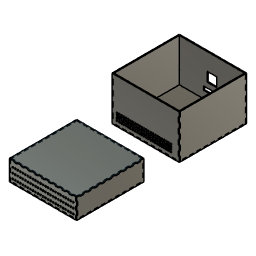
Boite projetV2 v3 (Autodesk Fusion 360 design; units mm, degrees)
Autodesk Fusion 360 part; units mm, degrees
(part 1 of 3)
sketch "Esquisse1" plane through (0, 0, 0) normal (0, 0, 1) x (1, 0, 0)
sketch "Esquisse2" plane through (0, 0, 0) normal (0, 0, 1) x (1, 0, 0)
  line L0 (0, 0) -> (200, 0)
  line L1 (200, 0) -> (200, 200)
  line L2 (200, 200) -> (0, 200)
  line L3 (0, 200) -> (0, 0)
  line L4 (0, 0) -> (10.5263, 0)
  line L5 (10.5263, 0) -> (10.5263, 3)
  line L6 (10.5263, 3) -> (0, 3)
  line L7 (0, 3) -> (0, 0)
  line L8 (10.5263, 0) -> (21.0526, 0)
  line L9 (21.0526, 0) -> (21.0526, 3)
  line L10 (21.0526, 3) -> (10.5263, 3)
  line L11 (10.5263, 3) -> (10.5263, 0)
  line L12 (21.0526, 0) -> (31.5789, 0)
  line L13 (31.5789, 0) -> (31.5789, 3)
  line L14 (31.5789, 3) -> (21.0526, 3)
  line L15 (21.0526, 3) -> (21.0526, 0)
  line L16 (31.5789, 0) -> (42.1053, 0)
  line L17 (42.1053, 0) -> (42.1053, 3)
  line L18 (42.1053, 3) -> (31.5789, 3)
  line L19 (31.5789, 3) -> (31.5789, 0)
  line L20 (42.1053, 0) -> (52.6316, 0)
  line L21 (52.6316, 0) -> (52.6316, 3)
  line L22 (52.6316, 3) -> (42.1053, 3)
  line L23 (42.1053, 3) -> (42.1053, 0)
  line L24 (52.6316, 0) -> (63.1579, 0)
  line L25 (63.1579, 0) -> (63.1579, 3)
  line L26 (63.1579, 3) -> (52.6316, 3)
  line L27 (52.6316, 3) -> (52.6316, 0)
  line L28 (63.1579, 0) -> (73.6842, 0)
  line L29 (73.6842, 0) -> (73.6842, 3)
  line L30 (73.6842, 3) -> (63.1579, 3)
  line L31 (63.1579, 3) -> (63.1579, 0)
  line L32 (73.6842, 0) -> (84.2105, 0)
  line L33 (84.2105, 0) -> (84.2105, 3)
  line L34 (84.2105, 3) -> (73.6842, 3)
  line L35 (73.6842, 3) -> (73.6842, 0)
  line L36 (84.2105, 0) -> (94.7368, 0)
  line L37 (94.7368, 0) -> (94.7368, 3)
  line L38 (94.7368, 3) -> (84.2105, 3)
  line L39 (84.2105, 3) -> (84.2105, 0)
  line L40 (94.7368, 0) -> (105.2632, 0)
  line L41 (105.2632, 0) -> (105.2632, 3)
  line L42 (105.2632, 3) -> (94.7368, 3)
  line L43 (94.7368, 3) -> (94.7368, 0)
  line L44 (105.2632, 0) -> (115.7895, 0)
  line L45 (115.7895, 0) -> (115.7895, 3)
  line L46 (115.7895, 3) -> (105.2632, 3)
  line L47 (105.2632, 3) -> (105.2632, 0)
  line L48 (115.7895, 0) -> (126.3158, 0)
  line L49 (126.3158, 0) -> (126.3158, 3)
  line L50 (126.3158, 3) -> (115.7895, 3)
  line L51 (115.7895, 3) -> (115.7895, 0)
  line L52 (126.3158, 0) -> (136.8421, 0)
  line L53 (136.8421, 0) -> (136.8421, 3)
  line L54 (136.8421, 3) -> (126.3158, 3)
  line L55 (126.3158, 3) -> (126.3158, 0)
  line L56 (136.8421, 0) -> (147.3684, 0)
  line L57 (147.3684, 0) -> (147.3684, 3)
  line L58 (147.3684, 3) -> (136.8421, 3)
  line L59 (136.8421, 3) -> (136.8421, 0)
  line L60 (147.3684, 0) -> (157.8947, 0)
  line L61 (157.8947, 0) -> (157.8947, 3)
  line L62 (157.8947, 3) -> (147.3684, 3)
  line L63 (147.3684, 3) -> (147.3684, 0)
  line L64 (157.8947, 0) -> (168.4211, 0)
  line L65 (168.4211, 0) -> (168.4211, 3)
  line L66 (168.4211, 3) -> (157.8947, 3)
  line L67 (157.8947, 3) -> (157.8947, 0)
  line L68 (168.4211, 0) -> (178.9474, 0)
  line L69 (178.9474, 0) -> (178.9474, 3)
  line L70 (178.9474, 3) -> (168.4211, 3)
  line L71 (168.4211, 3) -> (168.4211, 0)
  line L72 (178.9474, 0) -> (189.4737, 0)
  line L73 (189.4737, 0) -> (189.4737, 3)
  line L74 (189.4737, 3) -> (178.9474, 3)
  line L75 (178.9474, 3) -> (178.9474, 0)
  line L76 (189.4737, 0) -> (200, 0)
  line L77 (200, 0) -> (200, 3)
  line L78 (200, 3) -> (189.4737, 3)
  line L79 (189.4737, 3) -> (189.4737, 0)
  line L80 (0, 197) -> (10.5263, 197)
  line L81 (10.5263, 197) -> (10.5263, 200)
  line L82 (10.5263, 200) -> (0, 200)
  line L83 (0, 200) -> (0, 197)
  line L84 (10.5263, 197) -> (21.0526, 197)
  line L85 (21.0526, 197) -> (21.0526, 200)
  line L86 (21.0526, 200) -> (10.5263, 200)
  line L87 (10.5263, 200) -> (10.5263, 197)
  line L88 (21.0526, 197) -> (31.5789, 197)
  line L89 (31.5789, 197) -> (31.5789, 200)
  line L90 (31.5789, 200) -> (21.0526, 200)
  line L91 (21.0526, 200) -> (21.0526, 197)
  line L92 (31.5789, 197) -> (42.1053, 197)
  line L93 (42.1053, 197) -> (42.1053, 200)
  line L94 (42.1053, 200) -> (31.5789, 200)
  line L95 (31.5789, 200) -> (31.5789, 197)
  line L96 (42.1053, 197) -> (52.6316, 197)
  line L97 (52.6316, 197) -> (52.6316, 200)
  line L98 (52.6316, 200) -> (42.1053, 200)
  line L99 (42.1053, 200) -> (42.1053, 197)
  line L100 (52.6316, 197) -> (63.1579, 197)
  line L101 (63.1579, 197) -> (63.1579, 200)
  line L102 (63.1579, 200) -> (52.6316, 200)
  line L103 (52.6316, 200) -> (52.6316, 197)
  line L104 (63.1579, 197) -> (73.6842, 197)
  line L105 (73.6842, 197) -> (73.6842, 200)
  line L106 (73.6842, 200) -> (63.1579, 200)
  line L107 (63.1579, 200) -> (63.1579, 197)
  line L108 (73.6842, 197) -> (84.2105, 197)
  line L109 (84.2105, 197) -> (84.2105, 200)
  line L110 (84.2105, 200) -> (73.6842, 200)
  line L111 (73.6842, 200) -> (73.6842, 197)
  line L112 (84.2105, 197) -> (94.7368, 197)
  line L113 (94.7368, 197) -> (94.7368, 200)
  line L114 (94.7368, 200) -> (84.2105, 200)
  line L115 (84.2105, 200) -> (84.2105, 197)
  line L116 (94.7368, 197) -> (105.2632, 197)
  line L117 (105.2632, 197) -> (105.2632, 200)
  line L118 (105.2632, 200) -> (94.7368, 200)
  line L119 (94.7368, 200) -> (94.7368, 197)
  line L120 (105.2632, 197) -> (115.7895, 197)
  line L121 (115.7895, 197) -> (115.7895, 200)
  line L122 (115.7895, 200) -> (105.2632, 200)
  line L123 (105.2632, 200) -> (105.2632, 197)
  line L124 (115.7895, 197) -> (126.3158, 197)
  line L125 (126.3158, 197) -> (126.3158, 200)
  line L126 (126.3158, 200) -> (115.7895, 200)
  line L127 (115.7895, 200) -> (115.7895, 197)
  line L128 (126.3158, 197) -> (136.8421, 197)
  line L129 (136.8421, 197) -> (136.8421, 200)
  line L130 (136.8421, 200) -> (126.3158, 200)
  line L131 (126.3158, 200) -> (126.3158, 197)
  line L132 (136.8421, 197) -> (147.3684, 197)
  line L133 (147.3684, 197) -> (147.3684, 200)
  line L134 (147.3684, 200) -> (136.8421, 200)
  line L135 (136.8421, 200) -> (136.8421, 197)
  line L136 (147.3684, 197) -> (157.8947, 197)
  line L137 (157.8947, 197) -> (157.8947, 200)
  line L138 (157.8947, 200) -> (147.3684, 200)
  line L139 (147.3684, 200) -> (147.3684, 197)
  line L140 (157.8947, 197) -> (168.4211, 197)
  line L141 (168.4211, 197) -> (168.4211, 200)
  line L142 (168.4211, 200) -> (157.8947, 200)
  line L143 (157.8947, 200) -> (157.8947, 197)
  line L144 (168.4211, 197) -> (178.9474, 197)
  line L145 (178.9474, 197) -> (178.9474, 200)
  line L146 (178.9474, 200) -> (168.4211, 200)
  line L147 (168.4211, 200) -> (168.4211, 197)
  line L148 (178.9474, 197) -> (189.4737, 197)
  line L149 (189.4737, 197) -> (189.4737, 200)
  line L150 (189.4737, 200) -> (178.9474, 200)
  line L151 (178.9474, 200) -> (178.9474, 197)
  line L152 (189.4737, 197) -> (200, 197)
  line L153 (200, 197) -> (200, 200)
  line L154 (200, 200) -> (189.4737, 200)
  line L155 (189.4737, 200) -> (189.4737, 197)
  line L156 (0, 0) -> (3, 0)
  line L157 (3, 0) -> (3, 10.5263)
  line L158 (3, 10.5263) -> (0, 10.5263)
  line L159 (0, 10.5263) -> (0, 0)
  line L160 (197, 10.5263) -> (197, 0)
  line L161 (197, 0) -> (200, 0)
  line L162 (200, 0) -> (200, 10.5263)
  line L163 (200, 10.5263) -> (197, 10.5263)
  line L164 (0, 21.0526) -> (0, 10.5263)
  line L165 (0, 10.5263) -> (3, 10.5263)
  line L166 (3, 10.5263) -> (3, 21.0526)
  line L167 (3, 21.0526) -> (0, 21.0526)
  line L168 (197, 21.0526) -> (197, 10.5263)
  line L169 (197, 10.5263) -> (200, 10.5263)
  line L170 (200, 10.5263) -> (200, 21.0526)
  line L171 (200, 21.0526) -> (197, 21.0526)
  line L172 (0, 31.5789) -> (0, 21.0526)
  line L173 (0, 21.0526) -> (3, 21.0526)
  line L174 (3, 21.0526) -> (3, 31.5789)
  line L175 (3, 31.5789) -> (0, 31.5789)
  line L176 (197, 31.5789) -> (197, 21.0526)
  line L177 (197, 21.0526) -> (200, 21.0526)
  line L178 (200, 21.0526) -> (200, 31.5789)
  line L179 (200, 31.5789) -> (197, 31.5789)
  line L180 (0, 42.1053) -> (0, 31.5789)
  line L181 (0, 31.5789) -> (3, 31.5789)
  line L182 (3, 31.5789) -> (3, 42.1053)
  line L183 (3, 42.1053) -> (0, 42.1053)
  line L184 (197, 42.1053) -> (197, 31.5789)
  line L185 (197, 31.5789) -> (200, 31.5789)
  line L186 (200, 31.5789) -> (200, 42.1053)
  line L187 (200, 42.1053) -> (197, 42.1053)
  line L188 (0, 52.6316) -> (0, 42.1053)
  line L189 (0, 42.1053) -> (3, 42.1053)
  line L190 (3, 42.1053) -> (3, 52.6316)
  line L191 (3, 52.6316) -> (0, 52.6316)
  line L192 (197, 52.6316) -> (197, 42.1053)
  line L193 (197, 42.1053) -> (200, 42.1053)
  line L194 (200, 42.1053) -> (200, 52.6316)
  line L195 (200, 52.6316) -> (197, 52.6316)
  line L196 (0, 63.1579) -> (0, 52.6316)
  line L197 (0, 52.6316) -> (3, 52.6316)
  line L198 (3, 52.6316) -> (3, 63.1579)
  line L199 (3, 63.1579) -> (0, 63.1579)
  line L200 (197, 63.1579) -> (197, 52.6316)
  line L201 (197, 52.6316) -> (200, 52.6316)
  line L202 (200, 52.6316) -> (200, 63.1579)
  line L203 (200, 63.1579) -> (197, 63.1579)
  line L204 (0, 73.6842) -> (0, 63.1579)
  line L205 (0, 63.1579) -> (3, 63.1579)
  line L206 (3, 63.1579) -> (3, 73.6842)
  line L207 (3, 73.6842) -> (0, 73.6842)
  line L208 (197, 73.6842) -> (197, 63.1579)
  line L209 (197, 63.1579) -> (200, 63.1579)
  line L210 (200, 63.1579) -> (200, 73.6842)
  line L211 (200, 73.6842) -> (197, 73.6842)
  line L212 (0, 84.2105) -> (0, 73.6842)
  line L213 (0, 73.6842) -> (3, 73.6842)
  line L214 (3, 73.6842) -> (3, 84.2105)
  line L215 (3, 84.2105) -> (0, 84.2105)
  line L216 (197, 84.2105) -> (197, 73.6842)
  line L217 (197, 73.6842) -> (200, 73.6842)
  line L218 (200, 73.6842) -> (200, 84.2105)
  line L219 (200, 84.2105) -> (197, 84.2105)
  line L220 (0, 94.7368) -> (0, 84.2105)
  line L221 (0, 84.2105) -> (3, 84.2105)
  line L222 (3, 84.2105) -> (3, 94.7368)
  line L223 (3, 94.7368) -> (0, 94.7368)
  line L224 (197, 94.7368) -> (197, 84.2105)
  line L225 (197, 84.2105) -> (200, 84.2105)
  line L226 (200, 84.2105) -> (200, 94.7368)
  line L227 (200, 94.7368) -> (197, 94.7368)
  line L228 (0, 105.2632) -> (0, 94.7368)
  line L229 (0, 94.7368) -> (3, 94.7368)
  line L230 (3, 94.7368) -> (3, 105.2632)
  line L231 (3, 105.2632) -> (0, 105.2632)
  line L232 (197, 105.2632) -> (197, 94.7368)
  line L233 (197, 94.7368) -> (200, 94.7368)
  line L234 (200, 94.7368) -> (200, 105.2632)
  line L235 (200, 105.2632) -> (197, 105.2632)
  line L236 (0, 115.7895) -> (0, 105.2632)
  line L237 (0, 105.2632) -> (3, 105.2632)
  line L238 (3, 105.2632) -> (3, 115.7895)
  line L239 (3, 115.7895) -> (0, 115.7895)
  line L240 (197, 115.7895) -> (197, 105.2632)
  line L241 (197, 105.2632) -> (200, 105.2632)
  line L242 (200, 105.2632) -> (200, 115.7895)
  line L243 (200, 115.7895) -> (197, 115.7895)
  line L244 (0, 126.3158) -> (0, 115.7895)
  line L245 (0, 115.7895) -> (3, 115.7895)
  line L246 (3, 115.7895) -> (3, 126.3158)
  line L247 (3, 126.3158) -> (0, 126.3158)
  line L248 (197, 126.3158) -> (197, 115.7895)
  line L249 (197, 115.7895) -> (200, 115.7895)
  line L250 (200, 115.7895) -> (200, 126.3158)
  line L251 (200, 126.3158) -> (197, 126.3158)
  line L252 (0, 136.8421) -> (0, 126.3158)
  line L253 (0, 126.3158) -> (3, 126.3158)
  line L254 (3, 126.3158) -> (3, 136.8421)
  line L255 (3, 136.8421) -> (0, 136.8421)
  line L256 (197, 136.8421) -> (197, 126.3158)
  line L257 (197, 126.3158) -> (200, 126.3158)
  line L258 (200, 126.3158) -> (200, 136.8421)
  line L259 (200, 136.8421) -> (197, 136.8421)
  line L260 (0, 147.3684) -> (0, 136.8421)
  line L261 (0, 136.8421) -> (3, 136.8421)
  line L262 (3, 136.8421) -> (3, 147.3684)
  line L263 (3, 147.3684) -> (0, 147.3684)
  line L264 (197, 147.3684) -> (197, 136.8421)
  line L265 (197, 136.8421) -> (200, 136.8421)
  line L266 (200, 136.8421) -> (200, 147.3684)
  line L267 (200, 147.3684) -> (197, 147.3684)
  line L268 (0, 157.8947) -> (0, 147.3684)
  line L269 (0, 147.3684) -> (3, 147.3684)
  line L270 (3, 147.3684) -> (3, 157.8947)
  line L271 (3, 157.8947) -> (0, 157.8947)
  line L272 (197, 157.8947) -> (197, 147.3684)
  line L273 (197, 147.3684) -> (200, 147.3684)
  line L274 (200, 147.3684) -> (200, 157.8947)
  line L275 (200, 157.8947) -> (197, 157.8947)
  line L276 (0, 168.4211) -> (0, 157.8947)
  line L277 (0, 157.8947) -> (3, 157.8947)
  line L278 (3, 157.8947) -> (3, 168.4211)
  line L279 (3, 168.4211) -> (0, 168.4211)
  line L280 (197, 168.4211) -> (197, 157.8947)
  line L281 (197, 157.8947) -> (200, 157.8947)
  line L282 (200, 157.8947) -> (200, 168.4211)
  line L283 (200, 168.4211) -> (197, 168.4211)
  line L284 (0, 178.9474) -> (0, 168.4211)
  line L285 (0, 168.4211) -> (3, 168.4211)
  line L286 (3, 168.4211) -> (3, 178.9474)
  line L287 (3, 178.9474) -> (0, 178.9474)
  line L288 (197, 178.9474) -> (197, 168.4211)
  line L289 (197, 168.4211) -> (200, 168.4211)
  line L290 (200, 168.4211) -> (200, 178.9474)
  line L291 (200, 178.9474) -> (197, 178.9474)
  line L292 (0, 189.4737) -> (0, 178.9474)
  line L293 (0, 178.9474) -> (3, 178.9474)
  line L294 (3, 178.9474) -> (3, 189.4737)
  line L295 (3, 189.4737) -> (0, 189.4737)
  line L296 (197, 189.4737) -> (197, 178.9474)
  line L297 (197, 178.9474) -> (200, 178.9474)
  line L298 (200, 178.9474) -> (200, 189.4737)
  line L299 (200, 189.4737) -> (197, 189.4737)
  line L300 (0, 200) -> (0, 189.4737)
  line L301 (0, 189.4737) -> (3, 189.4737)
  line L302 (3, 189.4737) -> (3, 200)
  line L303 (3, 200) -> (0, 200)
  line L304 (197, 200) -> (197, 189.4737)
  line L305 (197, 189.4737) -> (200, 189.4737)
  line L306 (200, 189.4737) -> (200, 200)
  line L307 (200, 200) -> (197, 200)
  dimension "d9" = 200
  dimension "d10" = 200
  dimension "d11" = 10.5263
  dimension "d12" = 3
  dimension "d15" = 10.5263
  dimension "d16" = 197
  dimension "d17" = 3
  dimension "d18" = 10.5263
  dimension "d21" = 197
  dimension "d22" = 10.5263
  constraint horizontal L0
  constraint vertical L1
  constraint horizontal L2
  constraint vertical L3
  constraint coincident L0.start L3.end
  constraint horizontal L4
  constraint vertical L5
  constraint horizontal L6
  constraint vertical L7
  constraint horizontal L156
  constraint vertical L157
  constraint horizontal L158
  constraint vertical L159
  measures "d9" distance of L0.start L0.end
  measures "d10" distance of L0.start L2.end
  measures "d11" distance of L0.start L4.end
  measures "d12" distance of L0.start L6.end
  measures "d17" distance of L0.start L156.end
  measures "d18" distance of L0.start L158.end
extrude "Extrusion1" add sketch "Esquisse2" along normal blind 3 contours L0 L5 L8 L9 L10 L11 L15 | L6 L10 L14 L18 L22 L26 L30 L34 L38 L42 L46 L50 L54 L58 L62 L66 L70 L74 L78 L80 L84 L88 L92 L96 L100 L104 L108 L112 L116 L120 L124 L128 L132 L136 L140 L144 L148 L152 L157 L160 L166 L168 L174 L176 L182 L184 L190 L192 L198 L200 L206 L208 L214 L216 L222 L224 L230 L232 L238 L240 L246 L248 L254 L256 L262 L264 L270 L272 L278 L280 L286 L288 L294 L296 L302 L304 | L3 L158 L164 L165 L166 L167 L173 | L0 L13 L16 L17 L18 L19 L23 | L3 L175 L180 L181 L182 L183 L189 | L0 L21 L24 L25 L26 L27 L31 | L3 L191 L196 L197 L198 L199 L205 | L0 L29 L32 L33 L34 L35 L39 | L3 L207 L212 L213 L214 L215 L221 | L0 L37 L40 L41 L42 L43 L47 | L3 L223 L228 L229 L230 L231 L237 | L0 L45 L48 L49 L50 L51 L55 | L3 L239 L244 L245 L246 L247 L253 | L0 L53 L56 L57 L58 L59 L63 | L3 L255 L260 L261 L262 L263 L269 | L0 L61 L64 L65 L66 L67 L71 | L3 L271 L276 L277 L278 L279 L285 | L0 L69 L72 L73 L74 L75 L79 | L3 L287 L292 L293 L294 L295 L301 | L1 L163 L168 L169 L170 L171 L177 | L2 L81 L84 L85 L86 L87 L91 | L1 L179 L184 L185 L186 L187 L193 | L2 L89 L92 L93 L94 L95 L99 | L1 L195 L200 L201 L202 L203 L209 | L2 L97 L100 L101 L102 L103 L107 | L1 L211 L216 L217 L218 L219 L225 | L2 L105 L108 L109 L110 L111 L115 | L1 L227 L232 L233 L234 L235 L241 | L2 L113 L116 L117 L118 L119 L123 | L1 L243 L248 L249 L250 L251 L257 | L2 L121 L124 L125 L126 L127 L131 | L1 L259 L264 L265 L266 L267 L273 | L2 L129 L132 L133 L134 L135 L139 | L1 L275 L280 L281 L282 L283 L289 | L2 L137 L140 L141 L142 L143 L147 | L1 L291 L296 L297 L298 L299 L305 | L2 L145 L148 L149 L150 L151 L155 makes body 1
ref_plane "Plan de construction1" through (184.2105, 0, 1.5) normal (0, -1, 0) x (1, 0, 0)
sketch "Esquisse3" plane through (0, 0, 0) normal (0, -1, 0) x (-1, 0, 0)
  line L0 (0, 0) -> (-200, 0)
  line L1 (-200, 0) -> (-200, -130)
  line L2 (-200, -130) -> (0, -130)
  line L3 (0, -130) -> (0, 0)
  dimension "d26" = 200
  dimension "d27" = 130
  constraint horizontal L0
  constraint vertical L1
  constraint horizontal L2
  constraint vertical L3
  constraint coincident L0.start L3.end
  measures "d26" distance of L0.start L0.end
  measures "d27" distance of L0.start L2.end
extrude "Extrusion2" add sketch "Esquisse3" against normal blind 3 separate body makes body 2
combine "Combiner1" operation cut target body 2 tool bodies 1 keep tools
sketch "Esquisse4" plane through (0, 0, 0) normal (0, -1, 0) x (1, 0, 0)
  line L0 (10.5263, 0) -> (10.5263, 3)
  line L1 (10.5263, 3) -> (21.0526, 3)
  line L2 (21.0526, 3) -> (21.0526, 0)
  line L3 (21.0526, 0) -> (31.5789, 0)
  line L4 (31.5789, 0) -> (31.5789, 3)
  line L5 (31.5789, 3) -> (42.1053, 3)
  line L6 (42.1053, 3) -> (42.1053, 0)
  line L7 (42.1053, 0) -> (52.6316, 0)
  line L8 (52.6316, 0) -> (52.6316, 3)
  line L9 (52.6316, 3) -> (63.1579, 3)
  line L10 (63.1579, 3) -> (63.1579, 0)
  line L11 (63.1579, 0) -> (73.6842, 0)
  line L12 (73.6842, 0) -> (73.6842, 3)
  line L13 (73.6842, 3) -> (84.2105, 3)
  line L14 (84.2105, 3) -> (84.2105, 0)
  line L15 (84.2105, 0) -> (94.7368, 0)
  line L16 (94.7368, 0) -> (94.7368, 3)
  line L17 (94.7368, 3) -> (105.2632, 3)
  line L18 (105.2632, 3) -> (105.2632, 0)
  line L19 (105.2632, 0) -> (115.7895, 0)
  line L20 (115.7895, 0) -> (115.7895, 3)
  line L21 (115.7895, 3) -> (126.3158, 3)
  line L22 (126.3158, 3) -> (126.3158, 0)
  line L23 (126.3158, 0) -> (136.8421, 0)
  line L24 (136.8421, 0) -> (136.8421, 3)
  line L25 (136.8421, 3) -> (147.3684, 3)
  line L26 (147.3684, 3) -> (147.3684, 0)
  line L27 (147.3684, 0) -> (157.8947, 0)
  line L28 (157.8947, 0) -> (157.8947, 3)
  line L29 (157.8947, 3) -> (168.4211, 3)
  line L30 (168.4211, 3) -> (168.4211, 0)
  line L31 (168.4211, 0) -> (178.9474, 0)
  line L32 (178.9474, 0) -> (178.9474, 3)
  line L33 (178.9474, 3) -> (189.4737, 3)
  line L34 (189.4737, 3) -> (189.4737, 0)
  line L35 (189.4737, 0) -> (200, 0)
  line L36 (200, 0) -> (200, 130)
  line L37 (200, 130) -> (0, 130)
  line L38 (0, 130) -> (0, 0)
  line L39 (0, 0) -> (10.5263, 0)
  line L40 (0, 0) -> (3, 0)
  line L41 (3, 0) -> (3, 14.4444)
  line L42 (3, 14.4444) -> (0, 14.4444)
  line L43 (0, 14.4444) -> (0, 0)
  line L44 (197, 14.4444) -> (197, 0)
  line L45 (197, 0) -> (200, 0)
  line L46 (200, 0) -> (200, 14.4444)
  line L47 (200, 14.4444) -> (197, 14.4444)
  line L48 (0, 28.8889) -> (0, 14.4444)
  line L49 (0, 14.4444) -> (3, 14.4444)
  line L50 (3, 14.4444) -> (3, 28.8889)
  line L51 (3, 28.8889) -> (0, 28.8889)
  line L52 (197, 28.8889) -> (197, 14.4444)
  line L53 (197, 14.4444) -> (200, 14.4444)
  line L54 (200, 14.4444) -> (200, 28.8889)
  line L55 (200, 28.8889) -> (197, 28.8889)
  line L56 (0, 43.3333) -> (0, 28.8889)
  line L57 (0, 28.8889) -> (3, 28.8889)
  line L58 (3, 28.8889) -> (3, 43.3333)
  line L59 (3, 43.3333) -> (0, 43.3333)
  line L60 (197, 43.3333) -> (197, 28.8889)
  line L61 (197, 28.8889) -> (200, 28.8889)
  line L62 (200, 28.8889) -> (200, 43.3333)
  line L63 (200, 43.3333) -> (197, 43.3333)
  line L64 (0, 57.7778) -> (0, 43.3333)
  line L65 (0, 43.3333) -> (3, 43.3333)
  line L66 (3, 43.3333) -> (3, 57.7778)
  line L67 (3, 57.7778) -> (0, 57.7778)
  line L68 (197, 57.7778) -> (197, 43.3333)
  line L69 (197, 43.3333) -> (200, 43.3333)
  line L70 (200, 43.3333) -> (200, 57.7778)
  line L71 (200, 57.7778) -> (197, 57.7778)
  line L72 (0, 72.2222) -> (0, 57.7778)
  line L73 (0, 57.7778) -> (3, 57.7778)
  line L74 (3, 57.7778) -> (3, 72.2222)
  line L75 (3, 72.2222) -> (0, 72.2222)
  line L76 (197, 72.2222) -> (197, 57.7778)
  line L77 (197, 57.7778) -> (200, 57.7778)
  line L78 (200, 57.7778) -> (200, 72.2222)
  line L79 (200, 72.2222) -> (197, 72.2222)
  line L80 (0, 86.6667) -> (0, 72.2222)
  line L81 (0, 72.2222) -> (3, 72.2222)
  line L82 (3, 72.2222) -> (3, 86.6667)
  line L83 (3, 86.6667) -> (0, 86.6667)
  line L84 (197, 86.6667) -> (197, 72.2222)
  line L85 (197, 72.2222) -> (200, 72.2222)
  line L86 (200, 72.2222) -> (200, 86.6667)
  line L87 (200, 86.6667) -> (197, 86.6667)
  line L88 (0, 101.1111) -> (0, 86.6667)
  line L89 (0, 86.6667) -> (3, 86.6667)
  line L90 (3, 86.6667) -> (3, 101.1111)
  line L91 (3, 101.1111) -> (0, 101.1111)
  line L92 (197, 101.1111) -> (197, 86.6667)
  line L93 (197, 86.6667) -> (200, 86.6667)
  line L94 (200, 86.6667) -> (200, 101.1111)
  line L95 (200, 101.1111) -> (197, 101.1111)
  line L96 (0, 115.5556) -> (0, 101.1111)
  line L97 (0, 101.1111) -> (3, 101.1111)
  line L98 (3, 101.1111) -> (3, 115.5556)
  line L99 (3, 115.5556) -> (0, 115.5556)
  line L100 (197, 115.5556) -> (197, 101.1111)
  line L101 (197, 101.1111) -> (200, 101.1111)
  line L102 (200, 101.1111) -> (200, 115.5556)
  line L103 (200, 115.5556) -> (197, 115.5556)
  line L104 (0, 130) -> (0, 115.5556)
  line L105 (0, 115.5556) -> (3, 115.5556)
  line L106 (3, 115.5556) -> (3, 130)
  line L107 (3, 130) -> (0, 130)
  line L108 (197, 130) -> (197, 115.5556)
  line L109 (197, 115.5556) -> (200, 115.5556)
  line L110 (200, 115.5556) -> (200, 130)
  line L111 (200, 130) -> (197, 130)
  dimension "d30" = 3
  dimension "d31" = 14.4444
  dimension "d34" = 197
  dimension "d35" = 14.4444
  constraint horizontal L40
  constraint vertical L41
  constraint horizontal L42
  constraint vertical L43
  constraint coincident L38.end L39.start
  measures "d30" distance of L38.end L40.end
  measures "d31" distance of L38.end L42.end
extrude "Extrusion3" cut sketch "Esquisse4" against normal blind 3 contours L38 L42 L48 L49 L50 L51 L57 | L38 L59 L64 L65 L66 L67 L73 | L38 L75 L80 L81 L82 L83 L89 | L38 L91 L96 L97 L98 L99 L105 | L36 L95 L100 L101 L102 L103 L109 | L36 L79 L84 L85 L86 L87 L93 | L36 L63 L68 L69 L70 L71 L77 | L36 L47 L52 L53 L54 L55 L61 bodies 2
ref_plane "Plan de construction2" through (121.0526, 100, 1.5) normal (0, -1, 0) x (1, 0, 0)
mirror "Symétrie miroir1" about plane through (121.0526, 100, 1.5) normal (0, -1, 0) of bodies 2 makes body 3
ref_plane "Plan de construction3" through (200, 1.5, 65) normal (1, 0, 0) x (0, 0, -1)
sketch "Esquisse5" plane through (200, 0, 0) normal (1, 0, 0) x (0, 1, 0)
  line L0 (0, 0) -> (200, 0)
  line L1 (200, 0) -> (200, 130)
  line L2 (200, 130) -> (0, 130)
  line L3 (0, 130) -> (0, 0)
  dimension "d41" = 200
  dimension "d42" = 130
  constraint horizontal L0
  constraint vertical L1
  constraint horizontal L2
  constraint vertical L3
  constraint coincident L0.start L3.end
  measures "d41" distance of L0.start L0.end
  measures "d42" distance of L0.start L2.end
extrude "Extrusion4" add sketch "Esquisse5" against normal blind 3 separate body makes body 4
combine "Combiner2" operation cut target body 4 tool bodies 2 3 1 keep tools
ref_plane "Plan de construction4" through (100, 163.1579, 1.5) normal (-1, 0, 0) x (0, -1, 0)
mirror "Symétrie miroir2" about plane through (100, 163.1579, 1.5) normal (-1, 0, 0) of bodies 4 makes body 5
sketch "Esquisse6" plane through (0, 0, 3) normal (0, 0, 1) x (-1, 0, 0)
  line L0 (-189.4737, -200) -> (-178.9474, -200)
  line L1 (-178.9474, -200) -> (-178.9474, -197)
  line L2 (-178.9474, -197) -> (-168.4211, -197)
  line L3 (-168.4211, -197) -> (-168.4211, -200)
  line L4 (-168.4211, -200) -> (-157.8947, -200)
  line L5 (-157.8947, -200) -> (-157.8947, -197)
  line L6 (-157.8947, -197) -> (-147.3684, -197)
  line L7 (-147.3684, -197) -> (-147.3684, -200)
  line L8 (-147.3684, -200) -> (-136.8421, -200)
  line L9 (-136.8421, -200) -> (-136.8421, -197)
  line L10 (-136.8421, -197) -> (-126.3158, -197)
  line L11 (-126.3158, -197) -> (-126.3158, -200)
  line L12 (-126.3158, -200) -> (-115.7895, -200)
  line L13 (-115.7895, -200) -> (-115.7895, -197)
  line L14 (-115.7895, -197) -> (-105.2632, -197)
  line L15 (-105.2632, -197) -> (-105.2632, -200)
  line L16 (-105.2632, -200) -> (-94.7368, -200)
  line L17 (-94.7368, -200) -> (-94.7368, -197)
  line L18 (-94.7368, -197) -> (-84.2105, -197)
  line L19 (-84.2105, -197) -> (-84.2105, -200)
  line L20 (-84.2105, -200) -> (-73.6842, -200)
  line L21 (-73.6842, -200) -> (-73.6842, -197)
  line L22 (-73.6842, -197) -> (-63.1579, -197)
  line L23 (-63.1579, -197) -> (-63.1579, -200)
  line L24 (-63.1579, -200) -> (-52.6316, -200)
  line L25 (-52.6316, -200) -> (-52.6316, -197)
  line L26 (-52.6316, -197) -> (-42.1053, -197)
  line L27 (-42.1053, -197) -> (-42.1053, -200)
  line L28 (-42.1053, -200) -> (-31.5789, -200)
  line L29 (-31.5789, -200) -> (-31.5789, -197)
  line L30 (-31.5789, -197) -> (-21.0526, -197)
  line L31 (-21.0526, -197) -> (-21.0526, -200)
  line L32 (-21.0526, -200) -> (-10.5263, -200)
  line L33 (-10.5263, -200) -> (-10.5263, -197)
  line L34 (-10.5263, -197) -> (-3, -197)
  line L35 (-3, -197) -> (-3, -189.4737)
  line L36 (-3, -189.4737) -> (0, -189.4737)
  line L37 (0, -189.4737) -> (0, -178.9474)
  line L38 (0, -178.9474) -> (-3, -178.9474)
  line L39 (-3, -178.9474) -> (-3, -168.4211)
  line L40 (-3, -168.4211) -> (0, -168.4211)
  line L41 (0, -168.4211) -> (0, -157.8947)
  line L42 (0, -157.8947) -> (-3, -157.8947)
  line L43 (-3, -157.8947) -> (-3, -147.3684)
  line L44 (-3, -147.3684) -> (0, -147.3684)
  line L45 (0, -147.3684) -> (0, -136.8421)
  line L46 (0, -136.8421) -> (-3, -136.8421)
  line L47 (-3, -136.8421) -> (-3, -126.3158)
  line L48 (-3, -126.3158) -> (0, -126.3158)
  line L49 (0, -126.3158) -> (0, -115.7895)
  line L50 (0, -115.7895) -> (-3, -115.7895)
  line L51 (-3, -115.7895) -> (-3, -105.2632)
  line L52 (-3, -105.2632) -> (0, -105.2632)
  line L53 (0, -105.2632) -> (0, -94.7368)
  line L54 (0, -94.7368) -> (-3, -94.7368)
  line L55 (-3, -94.7368) -> (-3, -84.2105)
  line L56 (-3, -84.2105) -> (0, -84.2105)
  line L57 (0, -84.2105) -> (0, -73.6842)
  line L58 (0, -73.6842) -> (-3, -73.6842)
  line L59 (-3, -73.6842) -> (-3, -63.1579)
  line L60 (-3, -63.1579) -> (0, -63.1579)
  line L61 (0, -63.1579) -> (0, -52.6316)
  line L62 (0, -52.6316) -> (-3, -52.6316)
  line L63 (-3, -52.6316) -> (-3, -42.1053)
  line L64 (-3, -42.1053) -> (0, -42.1053)
  line L65 (0, -42.1053) -> (0, -31.5789)
  line L66 (0, -31.5789) -> (-3, -31.5789)
  line L67 (-3, -31.5789) -> (-3, -21.0526)
  line L68 (-3, -21.0526) -> (0, -21.0526)
  line L69 (0, -21.0526) -> (0, -10.5263)
  line L70 (0, -10.5263) -> (-3, -10.5263)
  line L71 (-3, -10.5263) -> (-3, -3)
  line L72 (-3, -3) -> (-10.5263, -3)
  line L73 (-10.5263, -3) -> (-10.5263, 0)
  line L74 (-10.5263, 0) -> (-21.0526, 0)
  line L75 (-21.0526, 0) -> (-21.0526, -3)
  line L76 (-21.0526, -3) -> (-31.5789, -3)
  line L77 (-31.5789, -3) -> (-31.5789, 0)
  line L78 (-31.5789, 0) -> (-42.1053, 0)
  line L79 (-42.1053, 0) -> (-42.1053, -3)
  line L80 (-42.1053, -3) -> (-52.6316, -3)
  line L81 (-52.6316, -3) -> (-52.6316, 0)
  line L82 (-52.6316, 0) -> (-63.1579, 0)
  line L83 (-63.1579, 0) -> (-63.1579, -3)
  line L84 (-63.1579, -3) -> (-73.6842, -3)
  line L85 (-73.6842, -3) -> (-73.6842, 0)
  line L86 (-73.6842, 0) -> (-84.2105, 0)
  line L87 (-84.2105, 0) -> (-84.2105, -3)
  line L88 (-84.2105, -3) -> (-94.7368, -3)
  line L89 (-94.7368, -3) -> (-94.7368, 0)
  line L90 (-94.7368, 0) -> (-105.2632, 0)
  line L91 (-105.2632, 0) -> (-105.2632, -3)
  line L92 (-105.2632, -3) -> (-115.7895, -3)
  line L93 (-115.7895, -3) -> (-115.7895, 0)
  line L94 (-115.7895, 0) -> (-126.3158, 0)
  line L95 (-126.3158, 0) -> (-126.3158, -3)
  line L96 (-126.3158, -3) -> (-136.8421, -3)
  line L97 (-136.8421, -3) -> (-136.8421, 0)
  line L98 (-136.8421, 0) -> (-147.3684, 0)
  line L99 (-147.3684, 0) -> (-147.3684, -3)
  line L100 (-147.3684, -3) -> (-157.8947, -3)
  line L101 (-157.8947, -3) -> (-157.8947, 0)
  line L102 (-157.8947, 0) -> (-168.4211, 0)
  line L103 (-168.4211, 0) -> (-168.4211, -3)
  line L104 (-168.4211, -3) -> (-178.9474, -3)
  line L105 (-178.9474, -3) -> (-178.9474, 0)
  line L106 (-178.9474, 0) -> (-189.4737, 0)
  line L107 (-189.4737, 0) -> (-189.4737, -3)
  line L108 (-189.4737, -3) -> (-197, -3)
  line L109 (-197, -3) -> (-197, -10.5263)
  line L110 (-197, -10.5263) -> (-200, -10.5263)
  line L111 (-200, -10.5263) -> (-200, -21.0526)
  line L112 (-200, -21.0526) -> (-197, -21.0526)
  line L113 (-197, -21.0526) -> (-197, -31.5789)
  line L114 (-197, -31.5789) -> (-200, -31.5789)
  line L115 (-200, -31.5789) -> (-200, -42.1053)
  line L116 (-200, -42.1053) -> (-197, -42.1053)
  line L117 (-197, -42.1053) -> (-197, -52.6316)
  line L118 (-197, -52.6316) -> (-200, -52.6316)
  line L119 (-200, -52.6316) -> (-200, -63.1579)
  line L120 (-200, -63.1579) -> (-197, -63.1579)
  line L121 (-197, -63.1579) -> (-197, -73.6842)
  line L122 (-197, -73.6842) -> (-200, -73.6842)
  line L123 (-200, -73.6842) -> (-200, -84.2105)
  line L124 (-200, -84.2105) -> (-197, -84.2105)
  line L125 (-197, -84.2105) -> (-197, -94.7368)
  line L126 (-197, -94.7368) -> (-200, -94.7368)
  line L127 (-200, -94.7368) -> (-200, -105.2632)
  line L128 (-200, -105.2632) -> (-197, -105.2632)
  line L129 (-197, -105.2632) -> (-197, -115.7895)
  line L130 (-197, -115.7895) -> (-200, -115.7895)
  line L131 (-200, -115.7895) -> (-200, -126.3158)
  line L132 (-200, -126.3158) -> (-197, -126.3158)
  line L133 (-197, -126.3158) -> (-197, -136.8421)
  line L134 (-197, -136.8421) -> (-200, -136.8421)
  line L135 (-200, -136.8421) -> (-200, -147.3684)
  line L136 (-200, -147.3684) -> (-197, -147.3684)
  line L137 (-197, -147.3684) -> (-197, -157.8947)
  line L138 (-197, -157.8947) -> (-200, -157.8947)
  line L139 (-200, -157.8947) -> (-200, -168.4211)
  line L140 (-200, -168.4211) -> (-197, -168.4211)
  line L141 (-197, -168.4211) -> (-197, -178.9474)
  line L142 (-197, -178.9474) -> (-200, -178.9474)
  line L143 (-200, -178.9474) -> (-200, -189.4737)
  line L144 (-200, -189.4737) -> (-197, -189.4737)
  line L145 (-197, -189.4737) -> (-197, -197)
  line L146 (-197, -197) -> (-189.4737, -197)
  line L147 (-189.4737, -197) -> (-189.4737, -200)
  line L148 (0, 50) -> (-200, 50)
  line L149 (-200, 50) -> (-200, 250)
  line L150 (-200, 250) -> (0, 250)
  line L151 (0, 250) -> (0, 50)
  line L152 (-200, 50) -> (-189.4737, 50)
  line L153 (-189.4737, 50) -> (-189.4737, 53)
  line L154 (-189.4737, 53) -> (-200, 53)
  line L155 (-200, 53) -> (-200, 50)
  line L156 (-189.4737, 50) -> (-178.9474, 50)
  line L157 (-178.9474, 50) -> (-178.9474, 53)
  line L158 (-178.9474, 53) -> (-189.4737, 53)
  line L159 (-189.4737, 53) -> (-189.4737, 50)
  line L160 (-178.9474, 50) -> (-168.4211, 50)
  line L161 (-168.4211, 50) -> (-168.4211, 53)
  line L162 (-168.4211, 53) -> (-178.9474, 53)
  line L163 (-178.9474, 53) -> (-178.9474, 50)
  line L164 (-168.4211, 50) -> (-157.8947, 50)
  line L165 (-157.8947, 50) -> (-157.8947, 53)
  line L166 (-157.8947, 53) -> (-168.4211, 53)
  line L167 (-168.4211, 53) -> (-168.4211, 50)
  line L168 (-157.8947, 50) -> (-147.3684, 50)
  line L169 (-147.3684, 50) -> (-147.3684, 53)
  line L170 (-147.3684, 53) -> (-157.8947, 53)
  line L171 (-157.8947, 53) -> (-157.8947, 50)
  line L172 (-147.3684, 50) -> (-136.8421, 50)
  line L173 (-136.8421, 50) -> (-136.8421, 53)
  line L174 (-136.8421, 53) -> (-147.3684, 53)
  line L175 (-147.3684, 53) -> (-147.3684, 50)
  line L176 (-136.8421, 50) -> (-126.3158, 50)
  line L177 (-126.3158, 50) -> (-126.3158, 53)
  line L178 (-126.3158, 53) -> (-136.8421, 53)
  line L179 (-136.8421, 53) -> (-136.8421, 50)
  line L180 (-126.3158, 50) -> (-115.7895, 50)
  line L181 (-115.7895, 50) -> (-115.7895, 53)
  line L182 (-115.7895, 53) -> (-126.3158, 53)
  line L183 (-126.3158, 53) -> (-126.3158, 50)
  line L184 (-115.7895, 50) -> (-105.2632, 50)
  line L185 (-105.2632, 50) -> (-105.2632, 53)
  line L186 (-105.2632, 53) -> (-115.7895, 53)
  line L187 (-115.7895, 53) -> (-115.7895, 50)
  line L188 (-105.2632, 50) -> (-94.7368, 50)
  line L189 (-94.7368, 50) -> (-94.7368, 53)
  line L190 (-94.7368, 53) -> (-105.2632, 53)
  line L191 (-105.2632, 53) -> (-105.2632, 50)
  line L192 (-94.7368, 50) -> (-84.2105, 50)
  line L193 (-84.2105, 50) -> (-84.2105, 53)
  line L194 (-84.2105, 53) -> (-94.7368, 53)
  line L195 (-94.7368, 53) -> (-94.7368, 50)
  line L196 (-84.2105, 50) -> (-73.6842, 50)
  line L197 (-73.6842, 50) -> (-73.6842, 53)
  line L198 (-73.6842, 53) -> (-84.2105, 53)
  line L199 (-84.2105, 53) -> (-84.2105, 50)
  line L200 (-73.6842, 50) -> (-63.1579, 50)
  line L201 (-63.1579, 50) -> (-63.1579, 53)
  line L202 (-63.1579, 53) -> (-73.6842, 53)
  line L203 (-73.6842, 53) -> (-73.6842, 50)
  line L204 (-63.1579, 50) -> (-52.6316, 50)
  line L205 (-52.6316, 50) -> (-52.6316, 53)
  line L206 (-52.6316, 53) -> (-63.1579, 53)
  line L207 (-63.1579, 53) -> (-63.1579, 50)
  line L208 (-52.6316, 50) -> (-42.1053, 50)
  line L209 (-42.1053, 50) -> (-42.1053, 53)
  line L210 (-42.1053, 53) -> (-52.6316, 53)
  line L211 (-52.6316, 53) -> (-52.6316, 50)
  line L212 (-42.1053, 50) -> (-31.5789, 50)
  line L213 (-31.5789, 50) -> (-31.5789, 53)
  line L214 (-31.5789, 53) -> (-42.1053, 53)
  line L215 (-42.1053, 53) -> (-42.1053, 50)
  line L216 (-31.5789, 50) -> (-21.0526, 50)
  line L217 (-21.0526, 50) -> (-21.0526, 53)
  line L218 (-21.0526, 53) -> (-31.5789, 53)
  line L219 (-31.5789, 53) -> (-31.5789, 50)
  line L220 (-21.0526, 50) -> (-10.5263, 50)
  line L221 (-10.5263, 50) -> (-10.5263, 53)
  line L222 (-10.5263, 53) -> (-21.0526, 53)
  line L223 (-21.0526, 53) -> (-21.0526, 50)
  line L224 (-10.5263, 50) -> (0, 50)
  line L225 (0, 50) -> (0, 53)
  line L226 (0, 53) -> (-10.5263, 53)
  line L227 (-10.5263, 53) -> (-10.5263, 50)
  line L228 (-200, 247) -> (-189.4737, 247)
  line L229 (-189.4737, 247) -> (-189.4737, 250)
  line L230 (-189.4737, 250) -> (-200, 250)
  line L231 (-200, 250) -> (-200, 247)
  line L232 (-189.4737, 247) -> (-178.9474, 247)
  line L233 (-178.9474, 247) -> (-178.9474, 250)
  line L234 (-178.9474, 250) -> (-189.4737, 250)
  line L235 (-189.4737, 250) -> (-189.4737, 247)
  line L236 (-178.9474, 247) -> (-168.4211, 247)
  line L237 (-168.4211, 247) -> (-168.4211, 250)
  line L238 (-168.4211, 250) -> (-178.9474, 250)
  line L239 (-178.9474, 250) -> (-178.9474, 247)
  line L240 (-168.4211, 247) -> (-157.8947, 247)
  line L241 (-157.8947, 247) -> (-157.8947, 250)
  line L242 (-157.8947, 250) -> (-168.4211, 250)
  line L243 (-168.4211, 250) -> (-168.4211, 247)
  line L244 (-157.8947, 247) -> (-147.3684, 247)
  line L245 (-147.3684, 247) -> (-147.3684, 250)
  line L246 (-147.3684, 250) -> (-157.8947, 250)
  line L247 (-157.8947, 250) -> (-157.8947, 247)
  line L248 (-147.3684, 247) -> (-136.8421, 247)
  line L249 (-136.8421, 247) -> (-136.8421, 250)
  line L250 (-136.8421, 250) -> (-147.3684, 250)
  line L251 (-147.3684, 250) -> (-147.3684, 247)
  line L252 (-136.8421, 247) -> (-126.3158, 247)
  line L253 (-126.3158, 247) -> (-126.3158, 250)
  line L254 (-126.3158, 250) -> (-136.8421, 250)
  line L255 (-136.8421, 250) -> (-136.8421, 247)
  line L256 (-126.3158, 247) -> (-115.7895, 247)
  line L257 (-115.7895, 247) -> (-115.7895, 250)
  line L258 (-115.7895, 250) -> (-126.3158, 250)
  line L259 (-126.3158, 250) -> (-126.3158, 247)
  line L260 (-115.7895, 247) -> (-105.2632, 247)
  line L261 (-105.2632, 247) -> (-105.2632, 250)
  line L262 (-105.2632, 250) -> (-115.7895, 250)
  line L263 (-115.7895, 250) -> (-115.7895, 247)
  line L264 (-105.2632, 247) -> (-94.7368, 247)
  line L265 (-94.7368, 247) -> (-94.7368, 250)
  line L266 (-94.7368, 250) -> (-105.2632, 250)
  line L267 (-105.2632, 250) -> (-105.2632, 247)
  line L268 (-94.7368, 247) -> (-84.2105, 247)
  line L269 (-84.2105, 247) -> (-84.2105, 250)
  line L270 (-84.2105, 250) -> (-94.7368, 250)
  line L271 (-94.7368, 250) -> (-94.7368, 247)
  line L272 (-84.2105, 247) -> (-73.6842, 247)
  line L273 (-73.6842, 247) -> (-73.6842, 250)
  line L274 (-73.6842, 250) -> (-84.2105, 250)
  line L275 (-84.2105, 250) -> (-84.2105, 247)
  line L276 (-73.6842, 247) -> (-63.1579, 247)
  line L277 (-63.1579, 247) -> (-63.1579, 250)
  line L278 (-63.1579, 250) -> (-73.6842, 250)
  line L279 (-73.6842, 250) -> (-73.6842, 247)
  line L280 (-63.1579, 247) -> (-52.6316, 247)
  line L281 (-52.6316, 247) -> (-52.6316, 250)
  line L282 (-52.6316, 250) -> (-63.1579, 250)
  line L283 (-63.1579, 250) -> (-63.1579, 247)
  line L284 (-52.6316, 247) -> (-42.1053, 247)
  line L285 (-42.1053, 247) -> (-42.1053, 250)
  line L286 (-42.1053, 250) -> (-52.6316, 250)
  line L287 (-52.6316, 250) -> (-52.6316, 247)
  line L288 (-42.1053, 247) -> (-31.5789, 247)
  line L289 (-31.5789, 247) -> (-31.5789, 250)
  line L290 (-31.5789, 250) -> (-42.1053, 250)
  line L291 (-42.1053, 250) -> (-42.1053, 247)
  line L292 (-31.5789, 247) -> (-21.0526, 247)
  line L293 (-21.0526, 247) -> (-21.0526, 250)
  line L294 (-21.0526, 250) -> (-31.5789, 250)
  line L295 (-31.5789, 250) -> (-31.5789, 247)
  line L296 (-21.0526, 247) -> (-10.5263, 247)
  line L297 (-10.5263, 247) -> (-10.5263, 250)
  line L298 (-10.5263, 250) -> (-21.0526, 250)
  line L299 (-21.0526, 250) -> (-21.0526, 247)
  line L300 (-10.5263, 247) -> (0, 247)
  line L301 (0, 247) -> (0, 250)
  line L302 (0, 250) -> (-10.5263, 250)
  line L303 (-10.5263, 250) -> (-10.5263, 247)
  line L304 (-200, 50) -> (-197, 50)
  line L305 (-197, 50) -> (-197, 60.5263)
  line L306 (-197, 60.5263) -> (-200, 60.5263)
  line L307 (-200, 60.5263) -> (-200, 50)
  line L308 (-3, 50) -> (0, 50)
  line L309 (0, 50) -> (0, 60.5263)
  line L310 (0, 60.5263) -> (-3, 60.5263)
  line L311 (-3, 60.5263) -> (-3, 50)
  line L312 (-200, 60.5263) -> (-197, 60.5263)
  line L313 (-197, 60.5263) -> (-197, 71.0526)
  line L314 (-197, 71.0526) -> (-200, 71.0526)
  line L315 (-200, 71.0526) -> (-200, 60.5263)
  line L316 (-3, 60.5263) -> (0, 60.5263)
  line L317 (0, 60.5263) -> (0, 71.0526)
  line L318 (0, 71.0526) -> (-3, 71.0526)
  line L319 (-3, 71.0526) -> (-3, 60.5263)
  line L320 (-200, 71.0526) -> (-197, 71.0526)
  line L321 (-197, 71.0526) -> (-197, 81.5789)
  line L322 (-197, 81.5789) -> (-200, 81.5789)
  line L323 (-200, 81.5789) -> (-200, 71.0526)
  line L324 (-3, 71.0526) -> (0, 71.0526)
  line L325 (0, 71.0526) -> (0, 81.5789)
  line L326 (0, 81.5789) -> (-3, 81.5789)
  line L327 (-3, 81.5789) -> (-3, 71.0526)
  line L328 (-200, 81.5789) -> (-197, 81.5789)
  line L329 (-197, 81.5789) -> (-197, 92.1053)
  line L330 (-197, 92.1053) -> (-200, 92.1053)
  line L331 (-200, 92.1053) -> (-200, 81.5789)
  line L332 (-3, 81.5789) -> (0, 81.5789)
  line L333 (0, 81.5789) -> (0, 92.1053)
  line L334 (0, 92.1053) -> (-3, 92.1053)
  line L335 (-3, 92.1053) -> (-3, 81.5789)
  line L336 (-200, 92.1053) -> (-197, 92.1053)
  line L337 (-197, 92.1053) -> (-197, 102.6316)
  line L338 (-197, 102.6316) -> (-200, 102.6316)
  line L339 (-200, 102.6316) -> (-200, 92.1053)
  line L340 (-3, 92.1053) -> (0, 92.1053)
  line L341 (0, 92.1053) -> (0, 102.6316)
  line L342 (0, 102.6316) -> (-3, 102.6316)
  line L343 (-3, 102.6316) -> (-3, 92.1053)
  line L344 (-200, 102.6316) -> (-197, 102.6316)
  line L345 (-197, 102.6316) -> (-197, 113.1579)
  line L346 (-197, 113.1579) -> (-200, 113.1579)
  line L347 (-200, 113.1579) -> (-200, 102.6316)
  line L348 (-3, 102.6316) -> (0, 102.6316)
  line L349 (0, 102.6316) -> (0, 113.1579)
  line L350 (0, 113.1579) -> (-3, 113.1579)
  line L351 (-3, 113.1579) -> (-3, 102.6316)
  line L352 (-200, 113.1579) -> (-197, 113.1579)
  line L353 (-197, 113.1579) -> (-197, 123.6842)
  line L354 (-197, 123.6842) -> (-200, 123.6842)
  line L355 (-200, 123.6842) -> (-200, 113.1579)
  line L356 (-3, 113.1579) -> (0, 113.1579)
  line L357 (0, 113.1579) -> (0, 123.6842)
  line L358 (0, 123.6842) -> (-3, 123.6842)
  line L359 (-3, 123.6842) -> (-3, 113.1579)
  line L360 (-200, 123.6842) -> (-197, 123.6842)
  line L361 (-197, 123.6842) -> (-197, 134.2105)
  line L362 (-197, 134.2105) -> (-200, 134.2105)
  line L363 (-200, 134.2105) -> (-200, 123.6842)
  line L364 (-3, 123.6842) -> (0, 123.6842)
  line L365 (0, 123.6842) -> (0, 134.2105)
  line L366 (0, 134.2105) -> (-3, 134.2105)
  line L367 (-3, 134.2105) -> (-3, 123.6842)
  line L368 (-200, 134.2105) -> (-197, 134.2105)
  line L369 (-197, 134.2105) -> (-197, 144.7368)
  line L370 (-197, 144.7368) -> (-200, 144.7368)
  line L371 (-200, 144.7368) -> (-200, 134.2105)
  line L372 (-3, 134.2105) -> (0, 134.2105)
  line L373 (0, 134.2105) -> (0, 144.7368)
  line L374 (0, 144.7368) -> (-3, 144.7368)
  line L375 (-3, 144.7368) -> (-3, 134.2105)
  line L376 (-200, 144.7368) -> (-197, 144.7368)
  line L377 (-197, 144.7368) -> (-197, 155.2632)
  line L378 (-197, 155.2632) -> (-200, 155.2632)
  line L379 (-200, 155.2632) -> (-200, 144.7368)
  line L380 (-3, 144.7368) -> (0, 144.7368)
  line L381 (0, 144.7368) -> (0, 155.2632)
  line L382 (0, 155.2632) -> (-3, 155.2632)
  line L383 (-3, 155.2632) -> (-3, 144.7368)
  line L384 (-200, 155.2632) -> (-197, 155.2632)
  line L385 (-197, 155.2632) -> (-197, 165.7895)
  line L386 (-197, 165.7895) -> (-200, 165.7895)
  line L387 (-200, 165.7895) -> (-200, 155.2632)
  line L388 (-3, 155.2632) -> (0, 155.2632)
  line L389 (0, 155.2632) -> (0, 165.7895)
  line L390 (0, 165.7895) -> (-3, 165.7895)
  line L391 (-3, 165.7895) -> (-3, 155.2632)
  line L392 (-200, 165.7895) -> (-197, 165.7895)
  line L393 (-197, 165.7895) -> (-197, 176.3158)
  line L394 (-197, 176.3158) -> (-200, 176.3158)
  line L395 (-200, 176.3158) -> (-200, 165.7895)
  line L396 (-3, 165.7895) -> (0, 165.7895)
  line L397 (0, 165.7895) -> (0, 176.3158)
  line L398 (0, 176.3158) -> (-3, 176.3158)
  line L399 (-3, 176.3158) -> (-3, 165.7895)
  line L400 (-200, 176.3158) -> (-197, 176.3158)
  line L401 (-197, 176.3158) -> (-197, 186.8421)
  line L402 (-197, 186.8421) -> (-200, 186.8421)
  line L403 (-200, 186.8421) -> (-200, 176.3158)
  line L404 (-3, 176.3158) -> (0, 176.3158)
  line L405 (0, 176.3158) -> (0, 186.8421)
  line L406 (0, 186.8421) -> (-3, 186.8421)
  line L407 (-3, 186.8421) -> (-3, 176.3158)
  line L408 (-200, 186.8421) -> (-197, 186.8421)
  line L409 (-197, 186.8421) -> (-197, 197.3684)
  line L410 (-197, 197.3684) -> (-200, 197.3684)
  line L411 (-200, 197.3684) -> (-200, 186.8421)
  line L412 (-3, 186.8421) -> (0, 186.8421)
  line L413 (0, 186.8421) -> (0, 197.3684)
  line L414 (0, 197.3684) -> (-3, 197.3684)
  line L415 (-3, 197.3684) -> (-3, 186.8421)
  line L416 (-200, 197.3684) -> (-197, 197.3684)
  line L417 (-197, 197.3684) -> (-197, 207.8947)
  line L418 (-197, 207.8947) -> (-200, 207.8947)
  line L419 (-200, 207.8947) -> (-200, 197.3684)
  line L420 (-3, 197.3684) -> (0, 197.3684)
  line L421 (0, 197.3684) -> (0, 207.8947)
  line L422 (0, 207.8947) -> (-3, 207.8947)
  line L423 (-3, 207.8947) -> (-3, 197.3684)
  line L424 (-200, 207.8947) -> (-197, 207.8947)
  line L425 (-197, 207.8947) -> (-197, 218.4211)
  line L426 (-197, 218.4211) -> (-200, 218.4211)
  line L427 (-200, 218.4211) -> (-200, 207.8947)
  line L428 (-3, 207.8947) -> (0, 207.8947)
  line L429 (0, 207.8947) -> (0, 218.4211)
  line L430 (0, 218.4211) -> (-3, 218.4211)
  line L431 (-3, 218.4211) -> (-3, 207.8947)
  line L432 (-200, 218.4211) -> (-197, 218.4211)
  line L433 (-197, 218.4211) -> (-197, 228.9474)
  line L434 (-197, 228.9474) -> (-200, 228.9474)
  line L435 (-200, 228.9474) -> (-200, 218.4211)
  line L436 (-3, 218.4211) -> (0, 218.4211)
  line L437 (0, 218.4211) -> (0, 228.9474)
  line L438 (0, 228.9474) -> (-3, 228.9474)
  line L439 (-3, 228.9474) -> (-3, 218.4211)
  line L440 (-200, 228.9474) -> (-197, 228.9474)
  line L441 (-197, 228.9474) -> (-197, 239.4737)
  line L442 (-197, 239.4737) -> (-200, 239.4737)
  line L443 (-200, 239.4737) -> (-200, 228.9474)
  line L444 (-3, 228.9474) -> (0, 228.9474)
  line L445 (0, 228.9474) -> (0, 239.4737)
  line L446 (0, 239.4737) -> (-3, 239.4737)
  line L447 (-3, 239.4737) -> (-3, 228.9474)
  line L448 (-200, 239.4737) -> (-197, 239.4737)
  line L449 (-197, 239.4737) -> (-197, 250)
  line L450 (-197, 250) -> (-200, 250)
  line L451 (-200, 250) -> (-200, 239.4737)
  line L452 (-3, 239.4737) -> (0, 239.4737)
  line L453 (0, 239.4737) -> (0, 250)
  line L454 (0, 250) -> (-3, 250)
  line L455 (-3, 250) -> (-3, 239.4737)
  dimension "d48" = 200
  dimension "d49" = 200
  dimension "d50" = 10.5263
  dimension "d51" = 3
  dimension "d54" = 10.5263
  dimension "d55" = 197
  dimension "d56" = 3
  dimension "d57" = 10.5263
  dimension "d60" = 197
  dimension "d61" = 10.5263
  constraint horizontal L148
  constraint vertical L149
  constraint horizontal L150
  constraint vertical L151
  constraint horizontal L152
  constraint vertical L153
  constraint horizontal L154
  constraint vertical L155
  constraint horizontal L304
  constraint vertical L305
  constraint horizontal L306
  constraint vertical L307
  measures "d48" distance of L148.start L148.end
  measures "d49" distance of L148.start L150.end
  measures "d50" distance of L148.end L152.end
  measures "d51" distance of L148.end L154.end
  measures "d56" distance of L148.end L304.end
  measures "d57" distance of L148.end L306.end
extrude "Extrusion5" add sketch "Esquisse6" along normal blind 3 separate body contours L148 L217 L220 L221 L222 L223 L227 | L154 L158 L162 L166 L170 L174 L178 L182 L186 L190 L194 L198 L202 L206 L210 L214 L218 L222 L226 L228 L232 L236 L240 L244 L248 L252 L256 L260 L264 L268 L272 L276 L280 L284 L288 L292 L296 L300 L305 L311 L313 L319 L321 L327 L329 L335 L337 L343 L345 L351 L353 L359 L361 L367 L369 L375 L377 L383 L385 L391 L393 L399 L401 L407 L409 L415 L417 L423 L425 L431 L433 L439 L441 L447 L449 L455 | L151 L310 L316 L317 L318 L319 L324 | L148 L209 L212 L213 L214 L215 L219 | L151 L326 L332 L333 L334 L335 L340 | L148 L201 L204 L205 L206 L207 L211 | L151 L342 L348 L349 L350 L351 L356 | L148 L193 L196 L197 L198 L199 L203 | L151 L358 L364 L365 L366 L367 L372 | L148 L185 L188 L189 L190 L191 L195 | L151 L374 L380 L381 L382 L383 L388 | L148 L177 L180 L181 L182 L183 L187 | L151 L390 L396 L397 L398 L399 L404 | L148 L169 L172 L173 L174 L175 L179 | L151 L406 L412 L413 L414 L415 L420 | L148 L161 L164 L165 L166 L167 L171 | L151 L422 L428 L429 L430 L431 L436 | L148 L153 L156 L157 L158 L159 L163 | L151 L438 L444 L445 L446 L447 L452 | L149 L306 L312 L313 L314 L315 L320 | L150 L293 L296 L297 L298 L299 L303 | L149 L322 L328 L329 L330 L331 L336 | L150 L285 L288 L289 L290 L291 L295 | L149 L338 L344 L345 L346 L347 L352 | L150 L277 L280 L281 L282 L283 L287 | L149 L354 L360 L361 L362 L363 L368 | L150 L269 L272 L273 L274 L275 L279 | L149 L370 L376 L377 L378 L379 L384 | L150 L261 L264 L265 L266 L267 L271 | L149 L386 L392 L393 L394 L395 L400 | L150 L253 L256 L257 L258 L259 L263 | L149 L402 L408 L409 L410 L411 L416 | L150 L245 L248 L249 L250 L251 L255 | L149 L418 L424 L425 L426 L427 L432 | L150 L237 L240 L241 L242 L243 L247 | L149 L434 L440 L441 L442 L443 L448 | L150 L229 L232 L233 L234 L235 L239 makes body 6
ref_plane "Plan de construction5" through (200, -65.7895, 4.5) normal (1, 0, 0) x (0, 1, 0)
sketch "Esquisse7" plane through (200, 0, 0) normal (1, 0, 0) x (0, 1, 0)
  line L0 (-50, 3) -> (-250, 3)
  line L1 (-250, 3) -> (-250, 63)
  line L2 (-250, 63) -> (-50, 63)
  line L3 (-50, 63) -> (-50, 3)
  point P0 (-50, 3)
  dimension "d65" = 200
  dimension "d66" = 60
  constraint horizontal L0
  constraint vertical L1
  constraint horizontal L2
  constraint vertical L3
  constraint coincident P0 L0.start
  measures "d65" distance of P0 L0.end
  measures "d66" distance of P0 L2.end
extrude "Extrusion6" add sketch "Esquisse7" against normal blind 3 separate body makes body 7
combine "Combiner3" operation cut target body 7 tool bodies 6 keep tools